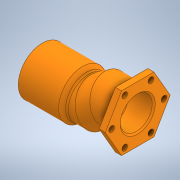
# Autodesk Inventor part: 22M_Standalone_Offset_Port_Hex_Female_Orange
Saved by Autodesk Inventor 2020 (Build 240168000, 168)
## iProperties
Created: 2021-06-18
Part Number: 22M_Standalone_Offset_Port_Hex_Female_Orange
Material: Generic
Document SubType Name: Modeling
Designer: Workshop
Density: 1 g/cm^3
Appearance: Orange
Author: Workshop
Autodesk Inventor part; units mm, degrees
ref_plane "YZ Plane" through (0, 0, 0) normal (1, 0, 0) x (0, 1, 0)
ref_plane "XZ Plane" through (0, 0, 0) normal (0, 1, 0) x (-1, 0, 0)
ref_plane "XY Plane" through (0, 0, 0) normal (0, 0, 1) x (1, 0, 0)
sketch "Sketch1" plane through (0, 0, 0) normal (0, 0, 1) x (1, 0, 0)
  line L0 (0, 0) -> (-11.591, 0)
  line L1 (-11.591, 0) -> (-19.9172, -6)
  line L2 (-19.9172, -6) -> (-25.1172, -6)
  dimension "d0" = 11.591
  dimension "d1" = 5.2
  dimension "d2" = 6
  dimension "d3" = 8.3262
  constraints: 6 end point, 1 horizontal, 1 parallel
  measures "d0" distance of L0.start L0.end
  measures "d1" distance of L1.end L2.end
  measures "d2" vertical distance of L0.start L1.end
  measures "d3" horizontal distance of L0.end L1.end
sketch "Sketch2" plane through (0, 0, 0) normal (1, 0, 0) x (0, 1, 0)
  circle A0 centre (0, 0) radius 11.625
  circle A1 centre (0, 0) radius 9.125
  dimension "d4" = 23.25
  dimension "d5" = 18.25
  constraints: 2 centre point, 2 coincident
  measures "d4" diameter of A0
  measures "d5" diameter of A1
sweep "Sweep1" add profiles "Sketch2" path "Sketch1"
sketch "Sketch5" plane through (0, 0, 0) normal (1, 0, 0) x (0, 0, -1)
  circle A0 centre (0, 0) radius 9.125 projected
  circle A1 centre (0, 0) radius 11.625 projected
  line L0 (9.2376, 16) -> (18.4752, 0)
  line L1 (18.4752, 0) -> (9.2376, -16)
  line L2 (9.2376, -16) -> (-9.2376, -16)
  line L3 (-9.2376, -16) -> (-18.4752, 0)
  line L4 (-18.4752, 0) -> (-9.2376, 16)
  line L5 (-9.2376, 16) -> (9.2376, 16)
  circle A2 centre (14.925, 0) radius 1.6
  circle A3 centre (7.4625, 12.9254) radius 1.6
  circle A4 centre (-7.4625, 12.9254) radius 1.6
  circle A5 centre (-14.925, 0) radius 1.6
  circle A6 centre (-7.4625, -12.9254) radius 1.6
  circle A7 centre (7.4625, -12.9254) radius 1.6
  point P0 (0, -16)
  dimension "d17" = 32
  dimension "d18" = 3.2
  dimension "d19" = 14.925
  dimension "d22" = 360
  constraints: 12 end point, 6 centre point, 1 coincident, 1 horizontal alignment, 1 midpoint, 1 vertical alignment, 26 other
  measures "d17" distance between parallel lines of L2 L5
  measures "d18" diameter of A2
  measures "d19" distance of point (0, 0) A2.centre
extrude "Extrusion1" add sketch "Sketch5" along normal blind 3.5 contours A1 | L0 L1 L2 L3 L4 L5
fillet "Fillet2" radius 0.8 1 edges at (0, -11.625, 0)
chamfer "Chamfer1" distance 0.875 angle 45 1 edges at (3.5, 0, 9.125)
sketch "Sketch6" plane through (0, 0, 0) normal (0, 0, 1) x (1, 0, 0)
  line L0 (-25.1172, -15.125) -> (-25.1172, 3.125) projected
  line L1 (-48.0149, -6) -> (-2.2195, -6)
  line L2 (-28.7511, -17.175) -> (-48.9388, -17.175)
  line L3 (-48.9388, -17.175) -> (-50.9388, -18.05)
  line L4 (-50.9388, -18.05) -> (-50.9388, -19.675)
  line L5 (-50.9388, -19.675) -> (-27.9388, -19.675)
  line L6 (-27.9388, -19.675) -> (-25.1172, -17.625)
  line L7 (-25.1172, 5.625) -> (-25.1172, -17.625) projected
  line L8 (-25.9295, -15.125) -> (-28.7511, -17.175)
  line L9 (-25.1172, -15.125) -> (-25.9295, -15.125)
  point P0 (0, 0)
  point P1 (-25.1172, -6)
  dimension "d32" = 22.35
  dimension "d33" = 23
  dimension "d34" = 2
  dimension "d35" = 0.875
  dimension "d36" = 2.5
  dimension "d37" = 126
  dimension "d38" = 2.5
  constraints: 16 end point, 3 perpendicular, 2 horizontal, 2 midpoint, 1 parallel
  measures "d32" diameter of L2 L1
  measures "d33" distance of L4.end L5.end
  measures "d34" horizontal distance of L2.end L3.end
  measures "d35" vertical distance of L2.end L3.end
  measures "d36" distance between parallel lines of L5 L2
  measures "d37" angle of L7 L6
  measures "d38" distance between parallel lines of L6 L8
revolve "Revolution2" add sketch "Sketch6" angle 360 about axis through (-48.0149, -6, 0) along (1, 0, 0)
fillet "Fillet4" radius 2 2 edges at (-25.1172, -6, -11.625) (-25.1172, -6, 11.625)
fillet "Fillet5" radius 2 1 edges at (-25.9295, 3.125, 0)
body "Solid1"
